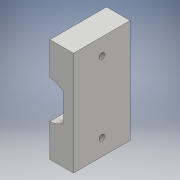
# Autodesk Inventor part: arm_2_case_bearing
Saved by Autodesk Inventor 2018 (Build 220112000, 112)
## iProperties
Created: 2018-02-05
Part Number: arm_2_case_bearing
Material: Genérico
Document SubType Name: Modeling
Designer: se_ma
Density: 1 g/cm^3
Appearance: Valor por defecto
Author: se_ma
Autodesk Inventor part; units mm, degrees
ref_plane "YZ Plane" through (0, 0, 0) normal (1, 0, 0) x (0, 1, 0)
ref_plane "XZ Plane" through (0, 0, 0) normal (0, 1, 0) x (-1, 0, 0)
ref_plane "XY Plane" through (0, 0, 0) normal (0, 0, 1) x (1, 0, 0)
sketch "Boceto1" plane through (0, 0, 0) normal (0, 1, 0) x (-1, 0, 0)
  line L0 (0, 0) -> (0, -55)
  line L1 (0, -55) -> (12.5, -55)
  line L2 (12.5, -55) -> (12.5, 0)
  line L3 (12.5, 0) -> (0, 0)
  dimension "d0" = 55
  dimension "d1" = 12.5
  constraints: 8 end point, 3 perpendicular, 1 vertical
  measures "d0" distance of L0.start L0.end
  measures "d1" distance of L0.end L1.end
extrude "Extrusión1" add sketch "Boceto1" along normal blind 30
sketch "Boceto2" plane through (0, 30, 0) normal (0, 1, 0) x (1, 0, 0)
  line L0 (-12.5, 27.5) -> (-12.5, 37.5)
  arc A0 (-12.5, 17.5) -> (-12.5, 37.5) centre (-12.5, 27.5) ccw
  line L1 (-12.5, 17.5) -> (-12.5, 27.5)
  line L2 (-12.5, 55) -> (-12.5, 0) projected
  point P0 (0, 0)
  dimension "d5" = 10
  constraints: 4 end point, 2 point on circle, 1 centre point, 1 coincident, 1 collinear
  measures "d5" distance of L0.start L0.end
extrude "Extrusión2" cut sketch "Boceto2" against normal blind 30
sketch "Boceto3" plane through (0, 30, 0) normal (0, 1, 0) x (1, 0, 0)
  line L0 (0, 0) -> (0, 55) projected
  line L1 (0, 27.5) -> (0, 20.5)
  line L2 (0, 20.5) -> (-5.3586, 20.5)
  arc A0 (-12.5, 17.5) -> (-12.5, 37.5) centre (-12.5, 27.5) ccw projected
  line L3 (-5.3586, 20.5) -> (-5.3586, 34.5)
  line L4 (-5.3586, 34.5) -> (0, 34.5)
  dimension "d8" = 7
  constraints: 8 end point, 3 perpendicular, 2 point on circle, 2 point on line, 1 midpoint
  measures "d8" distance of L1.start L1.end
extrude "Extrusión3" add sketch "Boceto3" against normal blind 2 contours L3 A0
sketch "Boceto4" plane through (-12.5, 0, 0) normal (-1, 0, 0) x (0, 0, 1)
  line L0 (-17.5, 30) -> (-17.5, 0) projected
  line L1 (-17.5, 15) -> (-37.5, 15)
  line L2 (-37.5, 0) -> (-37.5, 30) projected
  line L3 (-17.5, 15) -> (-17.5, 22.5)
  line L4 (-17.5, 22.5) -> (-37.5, 22.5)
  line L5 (-37.5, 22.5) -> (-37.5, 15)
  point P0 (0, 0)
  dimension "d11" = 7.5
  constraints: 8 end point, 2 midpoint, 2 perpendicular
  measures "d11" distance of L1.start L3.end
extrude "Extrusión4" add sketch "Boceto4" along normal blind 2
mirror "Simetría1" about plane through (-12.5, 22.5, -17.5) normal (0, 1, 0) of "Extrusión3"
mirror "Simetría2" about plane through (-12.5, 15, -37.5) normal (0, -1, 0) of "Extrusión3"
sketch "Boceto5" plane through (-14.5, 0, 0) normal (-1, 0, 0) x (0, 0, 1)
  line L0 (-17.5, 30) -> (-17.5, 22.5) projected
  line L1 (-17.5, 22.5) -> (-17.5, 15) projected
  line L2 (-17.5, 22.5) -> (-17.5, 15)
  line L3 (-37.5, 0) -> (-37.5, 15) projected
  line L4 (-17.5, 15) -> (-37.5, 15)
  line L5 (-37.5, 15) -> (-37.5, 22.5) projected
  line L6 (-37.5, 15) -> (-37.5, 22.5)
  line L7 (-37.5, 22.5) -> (-17.5, 22.5)
  point P0 (0, 0)
  constraints: 8 end point, 2 collinear, 2 perpendicular
extrude "Extrusión5" cut sketch "Boceto5" against normal blind 2
move faces "Desplazar1" translate (0, 6, 0) faces at (-4.4261, 17, -27.8685)
move faces "Desplazar2" translate (0, -8, 0) faces at (-4.4261, 15, -27.8685)
sketch "Boceto6" plane through (-12.5, 0, 0) normal (-1, 0, 0) x (0, 0, 1)
  line L0 (0, 30) -> (-55, 30) projected
  line L1 (-17.5, 30) -> (-17.5, 0) projected
  line L2 (0, 30) -> (-17.5, 30)
  line L3 (-8.75, 30) -> (-8.75, 15)
  line L4 (-37.5, 0) -> (-37.5, 30) projected
  line L5 (-55, 30) -> (-37.5, 30)
  line L6 (-46.25, 30) -> (-46.25, 15)
  circle A0 centre (-46.25, 15) radius 1.5
  circle A1 centre (-8.75, 15) radius 1.5
  point P0 (0, 0)
  dimension "d22" = 15
  dimension "d23" = 3
  dimension "d24" = 3
  constraints: 8 end point, 2 centre point, 2 coincident, 2 midpoint, 2 vertical, 1 horizontal, 1 perpendicular
  measures "d22" distance of L3.start L3.end
  measures "d23" diameter of A0
  measures "d24" diameter of A1
extrude "Extrusión6" cut sketch "Boceto6" against normal blind 12.5
